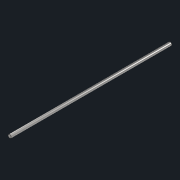
# Autodesk Inventor part: s_shaft
Saved by Autodesk Inventor 2022 (Build 260153000, 153)
## iProperties
Created: 2021-08-27
Part Number: s_shaft
Material: 鋼、炭素鋼
Document SubType Name: Modeling
Designer: Yuta Kage
Density: 7.85 g/cm^3
Appearance: 半つや出し
Author: Yuta Kage
Autodesk Inventor part; units mm, degrees
ref_plane "YZ Plane" through (0, 0, 0) normal (1, 0, 0) x (0, 1, 0)
ref_plane "XZ Plane" through (0, 0, 0) normal (0, 1, 0) x (-1, 0, 0)
ref_plane "XY Plane" through (0, 0, 0) normal (0, 0, 1) x (1, 0, 0)
sketch "スケッチ1" plane through (0, 0, 0) normal (0, 0, 1) x (1, 0, 0)
  circle A0 centre (0, 0) radius 3
  dimension "d0" = 6
  constraints: 1 centre point, 1 coincident
  measures "d0" diameter of A0
extrude "押し出し1" add sketch "スケッチ1" along normal mid plane 300
chamfer "面取り1" distance 0.5 angle 45 2 edges at (-3, 0, 150) (-3, 0, -150)
